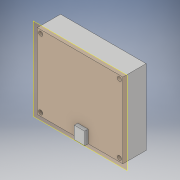
# Autodesk Inventor part: board_rev0
Saved by Autodesk Inventor 2018 (Build 220112000, 112)
## iProperties
Created: 2018-04-27
Part Number: board_rev0
Material: Generic
Document SubType Name: Modeling
Designer: rfabre
Density: 1 g/cm^3
Appearance: Default
Author: rfabre
Autodesk Inventor part; units mm, degrees
ref_plane "YZ Plane" through (0, 0, 0) normal (1, 0, 0) x (0, 1, 0)
ref_plane "XZ Plane" through (0, 0, 0) normal (0, 1, 0) x (-1, 0, 0)
ref_plane "XY Plane" through (0, 0, 0) normal (0, 0, 1) x (1, 0, 0)
sketch "Sketch1" plane through (0, 0, 0) normal (0, 0, 1) x (1, 0, 0)
  line L0 (0, 0) -> (62.2, 0)
  line L1 (62.2, 0) -> (62.2, 54.6)
  line L2 (62.2, 54.6) -> (0, 54.6)
  line L3 (0, 54.6) -> (0, 0)
  line L4 (1, 54.6) -> (1, 0) construction
  line L5 (0, 1) -> (62.2, 1) construction
  line L6 (61.2, 0) -> (61.2, 54.6) construction
  line L7 (0, 53.6) -> (62.2, 53.6) construction
  circle A0 centre (2.5, 52.1) radius 1.5
  circle A1 centre (59.7, 52.1) radius 1.5
  circle A2 centre (2.5, 2.5) radius 1.5
  circle A3 centre (59.7, 2.5) radius 1.5
  point P0 (33.2, 0)
  dimension "d0" = 62.2
  dimension "d1" = 54.6
  dimension "d2" = 29
  dimension "d3" = 1
  dimension "d4" = 1
  dimension "d5" = 1
  dimension "d6" = 1
  dimension "d7" = 3
  constraints: 16 end point, 9 point on line, 8 tangent, 5 perpendicular, 4 centre point, 3 equal radius, 2 parallel, 1 horizontal
  measures "d0" distance of L0.start L0.end
  measures "d1" distance of L2.end L0.start
  measures "d2" distance from line of L1 point (33.2, 0)
  measures "d3" distance of L2.end L4.start
  measures "d4" distance of L7.start L2.end
  measures "d5" distance of L1.end L6.end
  measures "d6" distance of L0.start L5.start
  measures "d7" diameter of A0
extrude "Extrusion1" add sketch "Sketch1" along normal blind 16.9
ref_plane "Work Plane1" through (0, 0, 16.9) normal (0, 0, 1) x (1, 0, 0)
sketch "Sketch2" plane through (0, 0, 16.9) normal (0, 0, 1) x (1, 0, 0)
  line L0 (0, 0) -> (62.2, 0) projected
  line L1 (29.4, 0) -> (37, 0)
  line L2 (37, 0) -> (37, 9.2)
  line L3 (37, 9.2) -> (29.4, 9.2)
  line L4 (29.4, 9.2) -> (29.4, 0)
  point P0 (33.2, 0)
  dimension "d11" = 29
  dimension "d12" = 7.6
  dimension "d13" = 9.2
  constraints: 8 end point, 2 parallel, 2 point on line, 1 horizontal, 1 midpoint, 1 perpendicular
  measures "d11" distance of point (33.2, 0) L0.end
  measures "d12" distance of L2.end L3.end
  measures "d13" distance of L1.end L2.end
extrude "Extrusion2" add sketch "Sketch2" along normal blind 2.5
equation "\"d4\" = d3"
equation "\"d5\" = d3"
equation "\"d6\" = d3"
body "Solid1"
